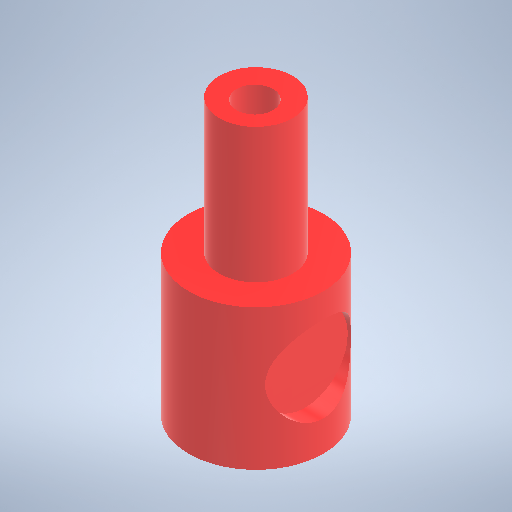
# Autodesk Inventor part: ventiltasse
Saved by Autodesk Inventor 2025 (Build 290162010, 162A)
## iProperties
Created: 2024-04-30
Part Number: ventiltasse
Material: Lead
Document SubType Name: Modeling
Designer: ffogue
Density: 11.34 g/cm^3
Appearance: Light Red
Author: ffogue
Autodesk Inventor part; units mm, degrees
ref_plane "XZ Plane" through (0, 0, 0) normal (0, 1, 0) x (-1, 0, 0)
ref_plane "XY Plane" through (0, 0, 0) normal (0, 0, 1) x (1, 0, 0)
sketch "Sketch1" plane through (0, 0, 0) normal (0, 1, 0) x (-1, 0, 0)
  line L0 (0, 0) -> (0, 22.5)
  line L1 (0, 22.5) -> (-3, 22.5)
  line L2 (-3, 22.5) -> (-3, 11.5)
  line L3 (-3, 11.5) -> (-5.5, 11.5)
  line L4 (-5.5, 11.5) -> (-5.5, 0)
  line L5 (-5.5, 0) -> (0, 0)
  point P0 (0, 11.25)
  point P1 (-1.5, 22.5)
  dimension "d0" = 11
  dimension "d1" = 6
  dimension "d2" = 11
  dimension "d3" = 11.5
  constraints: 12 end point, 5 perpendicular, 2 midpoint, 1 vertical
  measures "d0" diameter of L4 point (0, 11.25)
  measures "d1" diameter of L2 L0
  measures "d2" distance from line of L3 point (-1.5, 22.5)
  measures "d3" distance between parallel lines of L5 L3
revolve "Revolution1" add sketch "Sketch1" angle 360 about axis through (0, 0, 0) along (0, 0, 1)
sketch "Sketch2" plane through (0, 0, 0) normal (0, 0, -1) x (-1, 0, 0)
  circle A0 centre (0, 0) radius 5.5 projected
  constraints: 1 coincident
hole "Hole1" at (0, 0, 0) direction (0, 0, 1) diameter 6 depth 7
sketch "Sketch3" plane through (0, 0, 22.5) normal (0, 0, 1) x (1, 0, 0)
  point P0 (0, 0)
  point P1 (0.1316, -0.2274)
  dimension "d2" = 11
hole "Hole2" at (0.1316, -0.2274, 22.5) direction (0, 0, -1) diameter 3 depth 15.5
ref_plane "Work Plane1" through (5.5, 0, 0) normal (1, 0, 0) x (0, 1, 0)
sketch "Sketch4" plane through (5.5, 0, 0) normal (1, 0, 0) x (0, 1, 0)
  line L0 (5.5, 0) -> (-5.5, 0) projected
  point P0 (0, 0)
  point P1 (0, 6)
  dimension "d20" = 6
  constraints: 1 vertical alignment
  measures "d20" distance from line of L0 point (0, 6)
hole "Hole3" at (5.5, 0, 6) direction (-1, 0, 0) diameter 7 depth 1.5
body "Solid1"
